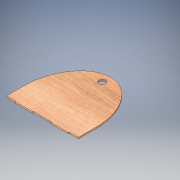
# Autodesk Inventor part: turretSidePlateTwo
Saved by Autodesk Inventor 2018 (Build 220112000, 112)
## iProperties
Created: 2019-02-27
Part Number: turretSidePlateTwo
Material: Generic
Document SubType Name: Modeling
Designer: snipe
Density: 1 g/cm^3
Appearance: Default
Author: snipe
Autodesk Inventor part; units mm, degrees
ref_plane "YZ Plane" through (0, 0, 0) normal (1, 0, 0) x (0, 1, 0)
ref_plane "XZ Plane" through (0, 0, 0) normal (0, 1, 0) x (-1, 0, 0)
ref_plane "XY Plane" through (0, 0, 0) normal (0, 0, 1) x (1, 0, 0)
sketch "Sketch1" plane through (0, 0, 0) normal (0, 1, 0) x (-1, 0, 0)
  line L0 (0, -234.315) -> (0, 339.09) projected
  line L1 (-213.36, 0) -> (213.36, 0) projected
  line L2 (213.36, 0) -> (-213.36, 0) projected
  line L3 (0, -234.315) -> (0, 339.09) projected
  line L4 (152.4, 254) -> (-152.4, 254)
  line L5 (-152.4, 254) -> (-152.4, 0)
  line L6 (152.4, 0) -> (152.4, 254)
  arc A0 (-152.4, 0) -> (152.4, 0) centre (0, 0) ccw
  line L7 (111.125, 254) -> (41.275, 254) construction
  line L8 (111.125, 257.175) -> (41.275, 257.175)
  line L9 (41.275, 250.825) -> (111.125, 250.825)
  arc A1 (111.125, 250.825) -> (111.125, 257.175) centre (111.125, 254) ccw
  arc A2 (41.275, 257.175) -> (41.275, 250.825) centre (41.275, 254) ccw
  line L10 (-41.275, 254) -> (-111.125, 254) construction
  line L11 (-41.275, 257.175) -> (-111.125, 257.175)
  line L12 (-111.125, 250.825) -> (-41.275, 250.825)
  arc A3 (-41.275, 250.825) -> (-41.275, 257.175) centre (-41.275, 254) ccw
  arc A4 (-111.125, 257.175) -> (-111.125, 250.825) centre (-111.125, 254) ccw
  circle A5 centre (0, 0) radius 14.2875
  point P0 (76.2, 254)
  point P1 (-76.2, 254)
  point P2 (0, -152.4)
  point P3 (114.3, 254)
  point P4 (38.1, 254)
  dimension "d2" = 69.85
  dimension "d3" = 6.35
  dimension "d4" = 69.85
  dimension "d5" = 6.35
  dimension "d7" = 76.2
  dimension "d8" = 304.8
  dimension "d9" = 76.2
  dimension "d10" = 28.575
  dimension "d11" = 406.4
  dimension "d15" = 76.2
  constraints: 22 end point, 12 point on circle, 10 tangent, 6 centre point, 4 point on line, 3 parallel, 2 coincident, 2 midpoint, 1 horizontal, 1 perpendicular
  measures "d2" distance of L7.start L7.end
  measures "d3" diameter of A2
  measures "d4" distance of L10.start L10.end
  measures "d5" diameter of A4
  measures "d7" distance from line of L0 point (76.2, 254)
  measures "d8" distance of L4.start L4.end
  measures "d9" distance from line of point (-76.2, 254) L0
  measures "d10" diameter of A5
  measures "d11" distance from line of L4 point (0, -152.4)
  measures "d15" distance of point (38.1, 254) point (114.3, 254)
extrude "Extrusion1" add sketch "Sketch1" along normal blind 6.35 contours A0 L1 A5 L0 | L0 A5 L1 A0 | L5 L4 A4 L12 A3 L0 A5 L1 | L1 A5 L0 L4 A2 L9 A1 L6 | A4 L11 A3 L4 | L4 A3 L12 A4 | A1 L9 A2 L4 | L4 A2 L8 A1
sketch "Sketch5" plane through (0, 6.35, 0) normal (0, 1, 0) x (1, 0, 0)
  circle A0 centre (0, 0) radius 14.2875 projected
  line L0 (-38.1, -254) -> (38.1, -254) projected
  arc A1 (38.1, -254) -> (41.275, -257.175) centre (41.275, -254) ccw projected
  line L1 (41.275, -257.175) -> (111.125, -257.175) projected
  arc A2 (111.125, -257.175) -> (114.3, -254) centre (111.125, -254) ccw projected
  line L2 (114.3, -254) -> (152.4, -254) projected
  line L3 (152.4, -254) -> (152.4, 0) projected
  arc A3 (152.4, 0) -> (-152.4, 0) centre (0, 0) ccw projected
  line L4 (-152.4, 0) -> (-152.4, -254) projected
  line L5 (-152.4, -254) -> (-114.3, -254) projected
  arc A4 (-114.3, -254) -> (-111.125, -257.175) centre (-111.125, -254) ccw projected
  line L6 (-111.125, -257.175) -> (-41.275, -257.175) projected
  arc A5 (-41.275, -257.175) -> (-38.1, -254) centre (-41.275, -254) ccw projected
  line L7 (-152.4, -254) -> (152.4, -254)
  line L8 (152.4, -254) -> (152.4, -177.8)
  line L9 (152.4, -177.8) -> (-152.4, -177.8)
  line L10 (-152.4, -177.8) -> (-152.4, -254)
  line L11 (-152.4, -177.8) -> (152.4, -177.8)
  line L12 (152.4, -177.8) -> (152.4, 0)
  line L13 (-152.4, 0) -> (-152.4, -177.8)
  arc A6 (152.4, 0) -> (-152.4, 0) centre (0, 0) ccw
  line L14 (-152.4, 0) -> (-152.4, -254) projected
  line L15 (-152.4, -177.8) -> (-152.4, 0) construction
  line L16 (-152.4, 0) -> (0, 152.4) construction
  line L17 (0, 152.4) -> (152.4, 0) construction
  line L18 (152.4, 0) -> (152.4, -177.8) construction
  line L19 (152.4, -254) -> (152.4, 0) projected
  spline S0 degree 4 poles (-152.4, -177.8) (-152.4, 0) (0, 152.4) (152.4, 0) (152.4, -177.8) knots 1 1 1 1 1 2 2 2 2 2
  dimension "d20" = 304.8
  dimension "d21" = 76.2
  constraints: 14 end point, 3 coincident, 3 parallel, 3 point on circle, 2 collinear, 2 horizontal, 2 perpendicular, 1 centre point, 3 other
  measures "d20" distance of L9.end L8.end
  measures "d21" distance of L8.end L7.end
extrude "Extrusion2" cut sketch "Sketch5" against normal blind 25.4 contours L4 A3 L3 S0
body "Solid1"
